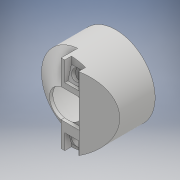
# Autodesk Inventor part: LightShield_olympus
Saved by Autodesk Inventor 2019 (Build 230136000, 136)
## iProperties
Created: 2016-05-01
Part Number: LightShield_olympus
Material: Generic
Document SubType Name: Modeling
Designer: Vervaeke-Lab
Density: 1 g/cm^3
Appearance: Default
Author: Vervaeke-Lab
Autodesk Inventor part; units mm, degrees
ref_plane "YZ Plane" through (0, 0, 0) normal (1, 0, 0) x (0, 1, 0)
sketch "Sketch1" plane through (0, 0, 0) normal (0, 1, 0) x (-1, 0, 0)
  circle A0 centre (0, 0) radius 19
  dimension "d0" = 38
  constraints: 1 centre point, 1 coincident
  measures "d0" diameter of A0
extrude "Extrusion-Main-Body" add sketch "Sketch1" along normal blind 25
sketch "Sketch2" plane through (0, 25, 0) normal (0, 1, 0) x (1, 0, 0)
  circle A0 centre (0, 0) radius 4.7
  dimension "d3" = 9.4
  constraints: 1 centre point, 1 coincident
  measures "d3" diameter of A0
extrude "Extrusion-Inner-Cylinder" cut sketch "Sketch2" against normal through all
sketch "Sketch3" plane through (0, 0, 0) normal (0, 0, 1) x (1, 0, 0)
  line L0 (4.7, 0) -> (-4.7, 0) projected
  line L1 (-4.7, 0) -> (-17.5501, 8.6675)
  line L2 (-4.7, 0) -> (10.8, 0) construction
  line L3 (-17.5501, 8.6675) -> (-17.5501, 25.6675)
  line L4 (0, 0) -> (-4.7, 0)
  line L5 (-17.5501, 25.6675) -> (0, 25.6675)
  line L6 (0, 25.6675) -> (0, 0)
  line L7 (-19, 0) -> (19, 0) projected
  dimension "d6" = 15.5
  dimension "d7" = 146
  constraints: 12 end point, 2 horizontal, 1 collinear, 1 equal length, 1 perpendicular, 1 vertical
  measures "d6" distance of L0.end L1.end
  measures "d7" angle of L2 L1
revolve "Revolution1" cut sketch "Sketch3" angle 360 about axis through (0, 25.6675, 0) along (0, -1, 0)
sketch "Sketch4" plane through (0, 0, 0) normal (0, -1, 0) x (1, 0, 0)
  line L0 (7.1, 24.2609) -> (0.3, 24.2609)
  line L1 (0.3, 24.2609) -> (0.3, 9.5)
  line L2 (0.3, 9.5) -> (7.1, 9.5)
  line L3 (7.1, 9.5) -> (7.1, 24.2609)
  line L4 (3.7, 9.5) -> (0.3, 9.5)
  point P0 (0, 0)
  dimension "d9" = 6.8
  dimension "d10" = 9.5
  dimension "d12" = 3.7
  constraints: 10 end point, 2 parallel, 1 collinear, 1 horizontal, 1 midpoint, 1 perpendicular
  measures "d9" distance of L1.end L2.end
  measures "d10" distance from line of point (0, 0) L2
  measures "d12" horizontal distance of point (0, 0) L4.start
extrude "Extrusion-Clamp-L" cut sketch "Sketch4" against normal blind 3.2
sketch "Sketch5" plane through (0, 0, 0) normal (0, -1, 0) x (1, 0, 0)
  line L0 (7.1, -21.5) -> (0.3, -21.5)
  line L1 (0.3, -21.5) -> (0.3, -11.5)
  line L2 (0.3, -11.5) -> (7.1, -11.5)
  line L3 (7.1, -11.5) -> (7.1, -21.5)
  line L4 (3.7, -11.5) -> (0.3, -11.5)
  point P0 (0, 0)
  dimension "d15" = 6.8
  dimension "d16" = 10
  dimension "d17" = 11.5
  dimension "d18" = 3.7
  constraints: 10 end point, 2 parallel, 2 perpendicular, 1 horizontal, 1 midpoint
  measures "d15" distance of L1.end L2.end
  measures "d16" distance of L0.end L1.end
  measures "d17" distance from line of point (0, 0) L2
  measures "d18" horizontal distance of point (0, 0) L4.start
extrude "Extrusion-Clamp-R" cut sketch "Sketch5" against normal blind 3.2
sketch "Sketch8" plane through (0, 0, 0) normal (0, 0, 1) x (1, 0, 0)
  line L0 (7.3313, 0) -> (19, 7.8707)
  line L1 (19, 0) -> (19, 25) projected
  line L2 (7.1, 0) -> (19, 0) projected
  line L3 (7.3313, 0) -> (19, 0)
  line L4 (19, 0) -> (19, 7.8707)
  point P0 (0, 0)
  dimension "d44" = 34
  constraints: 6 end point, 1 collinear, 1 perpendicular, 1 point on line
  measures "d44" angle of L0 L2
extrude "Extrusion-Back-Face" cut sketch "Sketch8" along normal through all both and the other way through all
sketch "Sketch9" plane through (0, 0, 0) normal (0, 0, 1) x (1, 0, 0)
  line L0 (-19, 0) -> (0.3, 0) projected
  line L1 (-7.0908, 0) -> (-19, 8.0329)
  line L2 (-19, 0) -> (-19, 25) projected
  line L3 (-7.0908, 0) -> (7.2743, 0) construction
  line L4 (-19, 8.0329) -> (-19, 0)
  line L5 (-19, 0) -> (-7.0908, 0)
  line L6 (0, -5) -> (0, 30) projected
  point P0 (0, 0)
  dimension "d34" = 146
  constraints: 8 end point, 2 collinear, 2 point on line, 1 equal length, 1 horizontal
  measures "d34" angle of L3 L1
revolve "Revolution-Front-Face" cut sketch "Sketch9" angle 180 mid plane about axis through (0, -10, 0) along (0, 1, 0)
ref_plane "Work Plane1" through (0, 0, 19) normal (0, 0, 1) x (1, 0, 0)
sketch "Sketch11" plane through (0, 0, 19) normal (0, 0, 1) x (1, 0, 0)
  line L0 (0, 0) -> (0, 8.0329) projected
  line L1 (0, 0) -> (-1.5, 0)
  line L2 (-7.0908, 0) -> (0, 0) projected
  line L3 (-1.5, 0) -> (-1.5, 8.0329)
  line L4 (0, 8.0329) -> (-19, 8.0329) projected
  line L5 (0, 8.0329) -> (0, 0)
  line L6 (0.3, 0) -> (0.3, 3.2) projected
  point P0 (0.2, 2.3)
  dimension "d38" = 1.5
  constraints: 6 end point, 2 point on line, 1 perpendicular, 1 vertical, 1 other
  measures "d38" distance of L0.start L1.end
extrude "Extrusion-Clamp-Support-L" add sketch "Sketch11" against normal up to next
ref_plane "Work Plane2" through (0, 0, -19) normal (0, 0, 1) x (1, 0, 0)
sketch "Sketch12" plane through (0, 0, -19) normal (0, 0, 1) x (1, 0, 0)
  line L0 (0, 0) -> (0, 8.0329) projected
  line L1 (0, 8.0329) -> (-19, 8.0329) projected
  line L2 (0, 0) -> (0, 8.0329)
  line L3 (0, 8.0329) -> (-1.5, 8.0329)
  line L4 (-17.5501, 8.6675) -> (17.5501, 8.6675) projected
  line L5 (-1.5, 8.0329) -> (-1.5, 0)
  line L6 (-7.0908, 0) -> (0, 0) projected
  line L7 (-1.5, 0) -> (0, 0)
  constraints: 8 end point, 1 collinear, 1 parallel, 1 perpendicular, 1 vertical
extrude "Extrusion-Clamp-Support-R" add sketch "Sketch12" along normal up to next
sketch "Sketch14" plane through (0, 0, 0) normal (0, -1, 0) x (1, 0, 0)
  circle A0 centre (0, 0) radius 19
  arc A1 (-1.5, 6.9303) -> (-1.5, -6.9303) centre (0, 0) ccw projected
  circle A2 centre (0, 0) radius 30.1648
  constraints: 2 centre point, 2 coincident
extrude "Extrusion14" cut sketch "Sketch14" against normal blind 25
sketch "Sketch23" plane through (7.1, 0, 9.5) normal (-1, 0, 0) x (0, 0, 1)
  line L0 (0, 0) -> (0, 3.2) projected
  line L1 (0, 3.2) -> (6.1, 3.2)
  line L2 (8.1236, 3.2) -> (0, 3.2) projected
  line L3 (0, 3.2) -> (0, 1.5)
  line L4 (0, 3.2) -> (1.7, 3.2) construction
  line L5 (0, 1.5) -> (6.1, 3.2)
  point P0 (-9.5, 0)
  dimension "d83" = 6.1
  dimension "d84" = 1.7
  dimension "d85" = 90
  constraints: 8 end point, 1 collinear, 1 horizontal, 1 perpendicular, 1 point on line
  measures "d83" distance of L0.end L1.end
  measures "d84" distance of L0.end L3.end
  measures "d85" angle of L3 L4
extrude "Extrusion-Clamp-Chamfer-L" add sketch "Sketch23" along normal blind 6.8
sketch "Sketch15" plane through (0.3, 0, -11.5) normal (1, 0, 0) x (0, 0, -1)
  line L0 (7.4976, 0) -> (0, 0) projected
  line L1 (0, 0) -> (6.1, 0)
  line L2 (6.1, 0) -> (6.1, 3.2)
  line L3 (7.4976, 3.2) -> (0, 3.2) projected
  line L4 (6.1, 3.2) -> (0, 1.5)
  line L5 (0, 0) -> (0, 3.2) projected
  line L6 (0, 1.5) -> (0, 3.2)
  line L7 (0, 3.2) -> (6.1, 3.2)
  point P0 (-11.5, 0)
  dimension "d54" = 6.1
  dimension "d55" = 1.7
  constraints: 10 end point, 3 point on line, 1 collinear, 1 perpendicular, 1 vertical
  measures "d54" distance of L0.end L1.end
  measures "d55" distance from line of L3 L4.end
extrude "Extrusion-Clamp-Chamfer-R" add sketch "Sketch15" along normal blind 7 contours L4 L5 L3
sketch "Sketch24" plane through (0.3, 3.2, 15.6) normal (0, -0.9632913, 0.2684582) x (1, 0, 0)
  circle A0 centre (3.4, -2.5325) radius 2.55
  line L0 (6.8, 0) -> (6.8, -6.3325) projected
  line L1 (6.8, -6.3325) -> (0, -6.3325) projected
  point P0 (-0.3, -15.8864)
  dimension "d88" = 5.1
  dimension "d89" = 3.4
  dimension "d90" = 3.8
  constraints: 1 centre point
  measures "d88" diameter of A0
  measures "d89" distance from line of L0 A0.centre
  measures "d90" distance from line of L1 A0.centre
extrude "Extrusion-Magnet-L" cut sketch "Sketch24" against normal blind 2
sketch "Sketch19" plane through (0.3, 1.5, -11.5) normal (0, -0.9632913, -0.2684582) x (1, 0, 0)
  line L0 (0, 0) -> (6.8, 0) projected
  line L1 (6.8, -6.3325) -> (0, -6.3325) projected
  circle A0 centre (3.4, -3.8) radius 2.55
  line L2 (0, -6.3325) -> (0, 0) projected
  point P0 (-0.3, 11.4805)
  point P1 (5.4784, -6.3325)
  dimension "d66" = 5.1
  dimension "d73" = 3.4
  dimension "d76" = 3.8
  constraints: 1 centre point
  measures "d66" diameter of A0
  measures "d73" distance from line of A0.centre L2
  measures "d76" distance from line of L0 A0.centre
extrude "Extrusion-Magnet-R" cut sketch "Sketch19" against normal blind 2
sketch "Sketch21" plane through (0, 0, 0) normal (0, -1, 0) x (1, 0, 0)
  line L0 (-1.5, -18.9407) -> (-1.5, -6.9303) projected
  line L1 (-1.5, -6.9303) -> (7.3313, -6.9303)
  line L2 (7.3313, -17.5286) -> (7.3313, 17.5286) projected
  arc A0 (-1.5, 6.9303) -> (-1.5, -6.9303) centre (0, 0) ccw projected
  line L3 (-1.5, 6.9303) -> (7.3313, 6.9303)
  line L4 (7.3313, 6.9303) -> (7.3313, -6.9303)
  line L5 (-1.5, 18.9407) -> (-1.5, 6.9303) projected
  arc A1 (-1.5, 6.9303) -> (-1.5, -6.9303) centre (0, 0) ccw
  constraints: 6 end point, 2 concentric, 2 horizontal, 2 point on circle, 1 centre point, 1 perpendicular, 1 point on line
extrude "Extrusion-Headbar-Top" cut sketch "Sketch21" against normal blind 1.75
body "Solid1"
